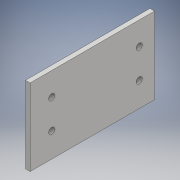
# Autodesk Inventor part: Part2
Saved by Autodesk Inventor 2018.3 (Build 223285000, 285)
## iProperties
Created: 2021-05-17
Part Number: Part2
Material: Generic
Document SubType Name: Modeling
Designer: Eugene
Density: 1 g/cm^3
Appearance: Default
Author: Eugene
Autodesk Inventor part; units mm, degrees
ref_plane "YZ Plane" through (0, 0, 0) normal (1, 0, 0) x (0, 1, 0)
ref_plane "XZ Plane" through (0, 0, 0) normal (0, 1, 0) x (-1, 0, 0)
ref_plane "XY Plane" through (0, 0, 0) normal (0, 0, 1) x (1, 0, 0)
sketch "Sketch1" plane through (0, 0, 0) normal (1, 0, 0) x (0, 1, 0)
  line L0 (0, 0) -> (81, 0)
  line L1 (81, 0) -> (81, -50)
  line L2 (81, -50) -> (0, -50)
  line L3 (0, -50) -> (0, 0)
  circle A0 centre (71, -15) radius 2
  circle A1 centre (71, -34) radius 2
  circle A2 centre (14, -15) radius 2
  circle A3 centre (14, -34) radius 2
  dimension "d0" = 81
  dimension "d1" = 50
  dimension "d2" = 4
  dimension "d3" = 15
  dimension "d4" = 4
  dimension "d5" = 16
  dimension "d6" = 4
  dimension "d7" = 15
  dimension "d8" = 4
  dimension "d9" = 57
  dimension "d11" = 10
  dimension "d12" = 57
  dimension "d13" = 10
  constraints: 8 end point, 4 centre point, 2 parallel, 1 horizontal, 1 perpendicular
  measures "d0" distance of L1.end L2.end
  measures "d1" distance of L0.end L1.end
  measures "d2" diameter of A0
  measures "d3" distance from line of L0 A0.centre
  measures "d4" diameter of A1
  measures "d5" distance from line of L2 A1.centre
  measures "d6" diameter of A2
  measures "d7" distance from line of L0 A2.centre
  measures "d8" diameter of A3
  measures "d9" distance of A3.centre A1.centre
  measures "d11" distance from line of L1 A1.centre
  measures "d12" distance of A2.centre A0.centre
  measures "d13" distance from line of L1 A0.centre
extrude "Extrusion1" add sketch "Sketch1" along normal blind 3
sketch "Sketch5" plane through (0, 81, 0) normal (0, 1, 0) x (1, 0, 0)
  circle A0 centre (7, 25) radius 4
  line L0 (0, 0) -> (3, 0) projected
  line L1 (3, 50) -> (3, 0) projected
  dimension "d26" = 8
  dimension "d27" = 25
  dimension "d28" = 4
  constraints: 1 centre point
  measures "d26" diameter of A0
  measures "d27" distance from line of L0 A0.centre
  measures "d28" distance from line of L1 A0.centre
extrude "Extrusion3" add sketch "Sketch5" against normal blind 81
sketch "Sketch8" plane through (0, 81, 0) normal (0, 1, 0) x (1, 0, 0)
  circle A0 centre (7, 25) radius 4
  line L0 (0, 0) -> (3, 0) projected
  line L1 (3, 50) -> (3, 25) projected
  point P0 (3, 29)
  dimension "d33" = 8
  dimension "d34" = 25
  dimension "d35" = 4
  constraints: 1 horizontal alignment, 1 other
  measures "d34" distance from line of L0 point (7, 25)
  measures "d35" distance from line of L1 point (7, 25)
extrude "Extrusion5" cut sketch "Sketch8" against normal blind 81
body "Solid1"
